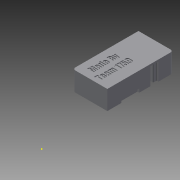
# Autodesk Inventor part: Positive Cap 535
Saved by Autodesk Inventor 2015 (Build 190159000, 159)
## iProperties
Created: 2015-01-23
Part Number: Positive Cap 535
Material: Generic
Document SubType Name: Modeling
Designer: pltwe4
Density: 1 g/cm^3
Appearance: Default
Author: pltwe4
Autodesk Inventor part; units mm, degrees
ref_plane "YZ Plane" through (0, 0, 0) normal (1, 0, 0) x (0, 1, 0)
ref_plane "XZ Plane" through (0, 0, 0) normal (0, 1, 0) x (-1, 0, 0)
ref_plane "XY Plane" through (0, 0, 0) normal (0, 0, 1) x (1, 0, 0)
sketch "Sketch1" plane through (0, 0, 0) normal (0, 1, 0) x (-1, 0, 0)
  line L0 (0, 0) -> (24.5364, 0)
  line L1 (24.5364, 0) -> (24.5364, -46.5582)
  line L2 (24.5364, -46.5582) -> (0, -46.5582)
  line L3 (0, -46.5582) -> (0, 0)
  dimension "d0" = 46.5582
  dimension "d1" = 24.5364
  constraints: 8 end point, 2 parallel, 1 horizontal, 1 perpendicular
  measures "d0" distance of L0.end L1.end
  measures "d1" distance of L1.end L2.end
extrude "Extrusion1" add sketch "Sketch1" along normal blind 13.5382
sketch "Sketch2" plane through (0, 0, 0) normal (0, -1, 0) x (1, 0, 0)
  point P0 (0, 0)
fillet "Fillet1" radius 1.905 1 edges at (-24.5364, 6.7691, -46.5582)
fillet "Fillet2" radius 1.905 1 edges at (0, 6.7691, 0)
sketch "Sketch3" plane through (0, 0, 0) normal (0, -1, 0) x (1, 0, 0)
  line L0 (-1.905, 0) -> (-24.5364, 0) projected
  arc A0 (0, -1.905) -> (-1.905, 0) centre (-1.905, -1.905) ccw projected
  line L1 (0, -46.5582) -> (0, -1.905) projected
  line L2 (-22.6314, -46.5582) -> (0, -46.5582) projected
  arc A1 (-24.5364, -44.6532) -> (-22.6314, -46.5582) centre (-22.6314, -44.6532) ccw projected
  line L3 (-24.5364, 0) -> (-24.5364, -44.6532) projected
  line L4 (-2.54, -2.54) -> (-21.9964, -2.54)
  line L5 (-21.9964, -44.0182) -> (-2.54, -44.0182)
  line L6 (0, -12.9032) -> (-4.445, -12.9032)
  line L7 (-4.445, -16.0782) -> (0, -16.0782)
  line L8 (-2.54, -44.0182) -> (-2.54, -18.6182)
  line L9 (-2.54, -10.3632) -> (-2.54, -2.54)
  line L10 (-4.445, -12.9032) -> (-4.445, -10.3632)
  line L11 (-4.445, -10.3632) -> (-2.54, -10.3632)
  line L12 (-4.445, -16.0782) -> (-4.445, -18.6182)
  line L13 (-4.445, -18.6182) -> (-2.54, -18.6182)
  line L14 (-21.9964, -10.3632) -> (-18.4404, -10.3632)
  line L15 (-18.4404, -10.3632) -> (-18.4404, -18.6182)
  line L16 (-18.4404, -18.6182) -> (-21.9964, -18.6182)
  line L17 (-21.9964, -2.54) -> (-21.9964, -10.3632)
  line L18 (-21.9964, -18.6182) -> (-21.9964, -44.0182)
  line L19 (0, -14.4907) -> (-5.2569, -14.4907) construction
  line L20 (-4.445, -11.6332) -> (-18.4404, -11.6332)
  line L21 (-4.445, -17.3482) -> (-18.4404, -17.3482)
  point P0 (0, 0)
  dimension "d7" = 2.54
  dimension "d9" = 2.54
  dimension "d11" = 3.175
  dimension "d13" = 4.445
  dimension "d14" = 2.54
  dimension "d15" = 2.54
  dimension "d16" = 2.54
  dimension "d17" = 2.54
  dimension "d20" = 2.54
  dimension "d21" = 6.096
  dimension "d22" = 2.54
  dimension "d37" = 32.0675
  constraints: 36 end point, 9 perpendicular, 7 parallel, 5 point on line, 4 horizontal, 2 collinear, 2 midpoint, 2 vertical, 1 other
  measures "d7" distance between parallel lines of L0 L4
  measures "d9" distance between parallel lines of L2 L5
  measures "d11" distance between parallel lines of L6 L7
  measures "d13" distance between parallel lines of L1 L10
  measures "d14" distance of L7.start L12.end
  measures "d15" distance of L6.end L10.end
  measures "d16" distance between parallel lines of L1 L8
  measures "d17" distance between parallel lines of L1 L9
  measures "d20" distance between parallel lines of L3 L18
  measures "d21" distance between parallel lines of L3 L15
  measures "d22" distance between parallel lines of L3 L17
  measures "d37" distance between parallel lines of L2 L19
extrude "Extrusion2" cut sketch "Sketch3" against normal blind 12.2682 contours L1 L7 L12 L21 L15 L20 L10 L6 | L20 L15 L14 L17 L4 L9 L11 L10 | L12 L13 L8 L5 L18 L16 L15 L21
sketch "Sketch4" plane through (0, 12.2682, 0) normal (0, -1, 0) x (1, 0, 0)
  line L0 (-4.5974, -23.6982) -> (-17.2974, -23.6982)
  line L1 (-17.2974, -23.6982) -> (-17.2974, -35.1282)
  line L2 (-17.2974, -35.1282) -> (-4.5974, -35.1282)
  line L3 (-4.5974, -35.1282) -> (-4.5974, -23.6982)
  line L4 (-2.54, -44.0182) -> (-21.9964, -44.0182) projected
  line L5 (-2.54, -18.6182) -> (-2.54, -44.0182) projected
  line L6 (-10.9474, -23.6982) -> (-10.9474, -35.1282) construction
  line L7 (-24.5364, 0) -> (-24.5364, -44.6532) construction
  line L8 (-22.6314, -46.5582) -> (0, -46.5582) construction
  point P0 (0, 0)
  dimension "d23" = 13.589
  dimension "d24" = 12.7
  dimension "d25" = 11.43
  dimension "d26" = 22.86
  constraints: 10 end point, 2 midpoint, 2 parallel, 1 horizontal, 1 perpendicular
  measures "d23" distance between parallel lines of L7 L6
  measures "d24" distance between parallel lines of L1 L3
  measures "d25" distance between parallel lines of L0 L2
  measures "d26" distance between parallel lines of L8 L0
extrude "Extrusion3" add sketch "Sketch4" along normal up to surface (12.2682 mm away)
sketch "Sketch5" plane through (-4.5974, 12.2682, -35.1282) normal (0, 0, -1) x (-1, 0, 0)
  line L0 (0, 0) -> (0, -12.2682) projected
  line L1 (12.7, 0) -> (12.7, -12.2682) projected
  line L2 (12.7, -12.2682) -> (0, -12.2682) projected
  arc A0 (8.2396, -6.5778) -> (4.4604, -6.5778) centre (6.35, -5.1816) ccw
  line L3 (6.35, -12.2682) -> (6.35, 0) construction
  line L4 (17.399, 0) -> (-2.0574, 0) construction
  line L5 (8.2396, -6.5778) -> (8.4707, -7.62)
  line L6 (8.4707, -7.62) -> (11.0107, -7.62)
  line L7 (11.0107, -7.62) -> (12.7, 0)
  line L8 (4.4604, -6.5778) -> (4.2293, -7.62)
  line L9 (4.2293, -7.62) -> (1.6893, -7.62)
  line L10 (1.6893, -7.62) -> (0, 0)
  point P0 (-4.5974, -12.2682)
  dimension "d29" = 7.0866
  dimension "d30" = 4.699
  dimension "d32" = 7.62
  dimension "d33" = 2.54
  dimension "d36" = 25
  constraints: 14 end point, 2 horizontal, 2 point on circle, 2 point on line, 1 centre point, 1 equal length, 1 midpoint, 1 parallel, 1 vertical, 2 other
  measures "d29" distance from line of L2 A0.centre
  measures "d30" diameter of A0
  measures "d32" distance between parallel lines of L4 L6
  measures "d33" distance of L5.end L6.end
  measures "d36" angle of L5 L8
extrude "Extrusion4" cut sketch "Sketch5" against normal up to surface (11.43 mm away)
sketch "Sketch6" plane through (0, 12.2682, 0) normal (0, -1, 0) x (1, 0, 0)
  line L0 (-4.445, -10.3632) -> (-4.445, -12.9032) projected
  line L1 (-4.445, -16.0782) -> (-4.445, -18.6182) projected
  line L2 (-18.4404, -18.6182) -> (-18.4404, -10.3632) projected
  line L3 (0, -12.9032) -> (0, -16.0782) projected
  line L4 (0, -16.0782) -> (-4.445, -16.0782) projected
  line L5 (-4.445, -12.9032) -> (0, -12.9032) projected
  line L6 (-4.445, -10.3632) -> (-18.4404, -10.3632)
  line L7 (-18.4404, -18.6182) -> (-4.445, -18.6182)
  line L8 (-1.27, -12.9032) -> (-1.27, -16.0782)
  point P0 (0, 0)
  dimension "d46" = 1.27
  constraints: 6 end point, 2 point on line, 1 horizontal, 1 parallel, 1 perpendicular
  measures "d46" distance between parallel lines of L8 L3
extrude "Extrusion5" cut sketch "Sketch6" against normal blind 0.635
sketch "Sketch7" plane through (0, 0, 0) normal (0, -1, 0) x (1, 0, 0)
  line L0 (0, -12.9032) -> (0, -1.905) projected
  line L1 (0, -1.905) -> (0, -46.5582) projected
  line L2 (0, -10.3632) -> (-0.635, -10.3632)
  line L3 (-1.27, -10.9982) -> (-1.27, -12.2682)
  arc A0 (-0.635, -10.3632) -> (-1.27, -10.9982) centre (-0.635, -10.9982) ccw
  line L4 (-1.905, -12.9032) -> (-4.445, -12.9032)
  line L5 (-4.445, -10.3632) -> (-4.445, -12.9032) projected
  arc A1 (-1.905, -12.9032) -> (-1.27, -12.2682) centre (-1.905, -12.2682) ccw
  line L6 (0, -10.3632) -> (0, -12.9032)
  line L7 (0, -12.9032) -> (-1.905, -12.9032)
  line L8 (-4.445, -12.9032) -> (0, -12.9032) projected
  point P0 (0, 0)
  point P1 (-1.27, -10.3632)
  point P2 (-1.27, -12.9032)
  dimension "d40" = 1.27
  dimension "d41" = 2.54
  dimension "d42" = 0.635
  dimension "d43" = 0.635
  constraints: 10 end point, 5 point on line, 5 tangent, 4 point on circle, 2 centre point, 2 collinear, 2 perpendicular, 1 parallel
  measures "d40" distance of L2.start point (-1.27, -10.363)
  measures "d41" distance of point (-1.27, -10.363) point (-1.27, -12.903)
  measures "d42" radius of A0
  measures "d43" radius of A1
extrude "Extrusion7" add sketch "Sketch6" against normal blind 0.635 contours L5 L3 L4 L8
extrude "Extrusion8" cut sketch "Sketch7" against normal up to surface (12.2682 mm away)
sketch "Sketch8" plane through (0, 0, -46.5582) normal (1, 0, 0) x (0, 0, -1)
  line L0 (-36.195, 0) -> (-36.195, 12.2682) projected
  line L1 (-30.48, 12.2682) -> (-36.195, 12.2682) projected
  line L2 (-30.48, 12.2682) -> (-30.48, 0) projected
  line L3 (0, 0) -> (-30.48, 0) projected
  line L4 (0, 0) -> (0, 13.5382) projected
  line L5 (-44.6532, 13.5382) -> (0, 13.5382) projected
  line L6 (-44.6532, 0) -> (-44.6532, 13.5382) projected
  line L7 (-36.195, 0) -> (-44.6532, 0) projected
  line L8 (-22.5397, 0) -> (-22.5397, 2.54)
  line L9 (-22.5397, 2.54) -> (-9.8397, 2.54)
  line L10 (-9.8397, 2.54) -> (-9.8397, 0)
  point P0 (-46.5582, 0)
  dimension "d51" = 2.54
  dimension "d52" = 12.7
  constraints: 6 end point, 2 perpendicular, 2 point on line, 1 vertical
  measures "d51" distance of L9.end L10.end
  measures "d52" distance of L8.end L9.end
extrude "Extrusion9" cut sketch "Sketch8" against normal blind 1.27 contours L8 L9 L10 L3
sketch "Sketch9" plane through (-4.5974, 12.2682, -35.1282) normal (0, 0, -1) x (-1, 0, 0)
  line L0 (12.7, 0) -> (11.0107, -7.62) projected
  line L1 (11.0107, -7.62) -> (8.4707, -7.62) projected
  line L2 (8.4707, -7.62) -> (8.2396, -6.5778) projected
  arc A0 (8.2396, -6.5778) -> (4.4604, -6.5778) centre (6.35, -5.1816) ccw projected
  line L3 (4.4604, -6.5778) -> (4.2293, -7.62) projected
  line L4 (4.2293, -7.62) -> (1.6893, -7.62) projected
  line L5 (1.6893, -7.62) -> (0, 0) projected
  line L6 (12.7, 0) -> (0, 0) projected
  line L7 (1.6893, -7.62) -> (11.0107, -7.62)
  line L8 (4.2293, -7.62) -> (1.6893, -7.62) projected
  point P0 (-4.5974, -12.2682)
  constraints: 2 end point, 1 collinear
extrude "Extrusion10" add sketch "Sketch9" along normal blind 2.54
mirror "Mirror1" about plane through (0, 0, -46.5582) normal (0, 0, -1) remove original yes
sketch "Sketch10" plane through (-24.5364, 13.5382, -93.1164) normal (0, 1, 0) x (1, 0, 0)
  arc A0 (24.5364, -1.905) -> (22.6314, 0) centre (22.6314, -1.905) ccw projected
  line L0 (0, 0) -> (22.6314, 0) projected
  line L1 (0, -44.6532) -> (0, 0) projected
  arc A1 (0, -44.6532) -> (1.905, -46.5582) centre (1.905, -44.6532) ccw projected
  line L2 (24.5364, -46.5582) -> (1.905, -46.5582) projected
  line L3 (24.5364, -1.905) -> (24.5364, -46.5582) projected
  line L4 (4.9657, -44.5516) -> (4.9657, -19.1516) construction
  line L5 (4.9657, -19.1516) -> (17.6657, -19.1516) construction
  line L6 (17.6657, -19.1516) -> (17.6657, -44.5516) construction
  line L7 (17.6657, -44.5516) -> (4.9657, -44.5516) construction
  line L8 (0, -44.6532) -> (0, 0) construction
  line L9 (24.5364, -1.905) -> (24.5364, -46.5582) construction
  line L10 (22.6314, 0) -> (0, 0) construction
  line L11 (24.5364, -46.5582) -> (1.905, -46.5582) construction
  line L12 (4.9657, -31.8516) -> (17.6657, -31.8516) construction
  line L13 (11.3157, -44.5516) -> (11.3157, -19.1516) construction
  line L14 (0, -22.3266) -> (24.5364, -22.3266) construction
  line L15 (11.3157, 0) -> (11.3157, -46.5582) construction
  line L16 (4.9657, -37.7102) -> (9.4107, -37.7102)
  line L17 (9.4107, -37.7102) -> (9.4107, -38.7218)
  line L18 (9.4107, -38.7218) -> (6.4094, -38.7218)
  line L19 (6.4094, -38.7218) -> (9.4107, -39.1271)
  line L20 (9.4107, -39.1271) -> (9.4107, -39.8405)
  line L21 (9.4107, -39.8405) -> (6.4764, -40.2626)
  line L22 (6.4764, -40.2626) -> (9.4107, -40.2659)
  line L23 (9.4107, -40.2659) -> (9.4107, -41.2775)
  line L24 (9.4107, -41.2775) -> (4.9657, -41.2775)
  line L25 (4.9657, -41.2775) -> (4.9657, -39.7802)
  spline S0 degree 2 poles (4.9657, -39.7802) (5.3643, -39.7166) (5.9103, -39.6429) knots 0 0 0 1 1 1
  line L26 (5.9103, -39.6429) -> (7.0425, -39.4788)
  line L27 (7.0425, -39.4788) -> (4.9657, -39.2175)
  line L28 (4.9657, -39.2175) -> (4.9657, -37.7102)
  line L29 (7.1765, -36.2866) -> (7.1765, -37.3283)
  line L30 (7.1765, -37.3283) -> (6.932, -37.3283)
  spline S1 degree 2 poles (6.932, -37.3283) (6.5099, -37.3283) (6.051, -37.134) (5.6993, -36.5445) (5.6993, -36.0755) knots 0 0 0 1 2 3 3 3
  spline S2 degree 2 poles (5.6993, -36.0755) (5.6993, -35.5128) (6.0979, -34.94) (6.6774, -34.8261) (7.5818, -34.8261) knots 0 0 0 1 2 3 3 3
  line L31 (7.5818, -34.8261) -> (9.4107, -34.8261)
  line L32 (9.4107, -34.8261) -> (9.4107, -35.9047)
  line L33 (9.4107, -35.9047) -> (9.0858, -35.9047)
  spline S3 degree 2 poles (9.0858, -35.9047) (9.2801, -36.0052) (9.4777, -36.3267) (9.4777, -36.5512) knots 0 0 0 1 2 2 2
  spline S4 degree 2 poles (9.4777, -36.5512) (9.4777, -36.8426) (9.1494, -37.3283) (8.5967, -37.3283) knots 0 0 0 1 2 2 2
  line L34 (8.5967, -37.3283) -> (8.2986, -37.3283)
  spline S5 degree 2 poles (8.2986, -37.3283) (7.89, -37.3283) (7.5918, -37.0704) (7.3942, -36.5579) knots 0 0 0 1 2 2 2
  spline S6 degree 2 poles (7.3942, -36.5579) (7.1798, -36.0119) (7.0324, -35.9348) (6.8047, -35.9348) knots 0 0 0 1 2 2 2
  spline S7 degree 2 poles (6.8047, -35.9348) (6.5199, -35.9348) (6.3458, -36.0186) (6.3458, -36.1191) knots 0 0 0 1 2 2 2
  spline S8 degree 2 poles (6.3458, -36.1191) (6.3458, -36.233) (6.4898, -36.2866) (6.7946, -36.2866) knots 0 0 0 1 2 2 2
  line L35 (6.7946, -36.2866) -> (7.1765, -36.2866)
  spline S9 degree 2 poles (7.6756, -35.9348) (7.8699, -36.2028) (8.1345, -36.2866) (8.3824, -36.2866) knots 0 0 0 1 2 2 2
  spline S10 degree 2 poles (8.3824, -36.2866) (8.6671, -36.2866) (8.8312, -36.2129) (8.8312, -36.1023) knots 0 0 0 1 2 2 2
  spline S11 degree 2 poles (8.8312, -36.1023) (8.8312, -35.9985) (8.7006, -35.9348) (8.4259, -35.9348) knots 0 0 0 1 2 2 2
  line L36 (8.4259, -35.9348) -> (7.6756, -35.9348)
  line L37 (4.9657, -31.9219) -> (9.4107, -31.9219)
  line L38 (9.4107, -31.9219) -> (9.4107, -33.0307)
  line L39 (9.4107, -33.0307) -> (9.1461, -33.0307)
  spline S12 degree 2 poles (9.1461, -33.0307) (9.3136, -33.1915) (9.4777, -33.5398) (9.4777, -33.7341) knots 0 0 0 1 2 2 2
  spline S13 degree 2 poles (9.4777, -33.7341) (9.4777, -33.992) (9.2064, -34.3705) (8.848, -34.4777) (8.446, -34.4777) knots 0 0 0 1 2 3 3 3
  line L40 (8.446, -34.4777) -> (6.7377, -34.4777)
  spline S14 degree 2 poles (6.7377, -34.4777) (6.319, -34.4777) (5.9672, -34.3705) (5.6993, -33.9853) (5.6993, -33.7207) knots 0 0 0 1 2 3 3 3
  spline S15 degree 2 poles (5.6993, -33.7207) (5.6993, -33.513) (5.8467, -33.1714) (5.9974, -33.0307) knots 0 0 0 1 2 2 2
  line L41 (5.9974, -33.0307) -> (4.9657, -33.0307)
  line L42 (4.9657, -33.0307) -> (4.9657, -31.9219)
  spline S16 degree 2 poles (6.6841, -33.0307) (6.4831, -33.0307) (6.3458, -33.101) (6.3458, -33.2015) knots 0 0 0 1 2 2 2
  spline S17 degree 2 poles (6.3458, -33.2015) (6.3458, -33.2987) (6.4697, -33.369) (6.6841, -33.369) knots 0 0 0 1 2 2 2
  line L43 (6.6841, -33.369) -> (8.4694, -33.369)
  spline S18 degree 2 poles (8.4694, -33.369) (8.6905, -33.369) (8.8312, -33.302) (8.8312, -33.2082) knots 0 0 0 1 2 2 2
  spline S19 degree 2 poles (8.8312, -33.2082) (8.8312, -33.101) (8.6738, -33.0307) (8.369, -33.0307) knots 0 0 0 1 2 2 2
  line L44 (8.369, -33.0307) -> (6.6841, -33.0307)
  line L45 (7.6521, -29.0111) -> (7.6521, -30.4481)
  line L46 (7.6521, -30.4481) -> (8.4393, -30.4481)
  spline S20 degree 2 poles (8.4393, -30.4481) (8.6872, -30.4481) (8.8312, -30.3777) (8.8312, -30.2739) knots 0 0 0 1 2 2 2
  spline S21 degree 2 poles (8.8312, -30.2739) (8.8312, -30.1466) (8.6403, -30.0629) (8.369, -30.0629) knots 0 0 0 1 2 2 2
  line L47 (8.369, -30.0629) -> (7.89, -30.0629)
  line L48 (7.89, -30.0629) -> (7.89, -29.0111)
  line L49 (7.89, -29.0111) -> (8.1579, -29.0111)
  spline S22 degree 2 poles (8.1579, -29.0111) (8.4962, -29.0111) (8.858, -29.0948) (9.27, -29.4097) (9.4777, -29.8887) (9.4777, -30.2538) knots 0 0 0 1 2 3 4 4 4
  spline S23 degree 2 poles (9.4777, -30.2538) (9.4777, -30.6055) (9.2734, -31.1415) (8.9183, -31.4429) (8.4929, -31.5568) (8.0876, -31.5568) knots 0 0 0 1 2 3 4 4 4
  line L50 (8.0876, -31.5568) -> (7.0224, -31.5568)
  spline S24 degree 2 poles (7.0224, -31.5568) (6.5467, -31.5568) (5.994, -31.2989) (5.6993, -30.7094) (5.6993, -30.3309) knots 0 0 0 1 2 3 3 3
  spline S25 degree 2 poles (5.6993, -30.3309) (5.6993, -29.8619) (6.0543, -29.2556) (6.6372, -29.0111) (7.1698, -29.0111) knots 0 0 0 1 2 3 3 3
  line L51 (7.1698, -29.0111) -> (7.6521, -29.0111)
  line L52 (7.0592, -30.1232) -> (6.7946, -30.1232)
  spline S26 degree 2 poles (6.7946, -30.1232) (6.5099, -30.1232) (6.3458, -30.1835) (6.3458, -30.2773) knots 0 0 0 1 2 2 2
  spline S27 degree 2 poles (6.3458, -30.2773) (6.3458, -30.3945) (6.4864, -30.4481) (6.7946, -30.4481) knots 0 0 0 1 2 2 2
  line L53 (6.7946, -30.4481) -> (7.0592, -30.4481)
  line L54 (7.0592, -30.4481) -> (7.0592, -30.1232)
  line L55 (4.9657, -27.6243) -> (4.9657, -26.472)
  spline S28 degree 2 poles (4.9657, -26.472) (4.9657, -25.9227) (5.1365, -25.36) (5.6557, -25.0149) (6.2319, -25.0149) knots 0 0 0 1 2 3 3 3
  spline S29 degree 2 poles (6.2319, -25.0149) (6.6204, -25.0149) (6.9286, -25.2595) (7.009, -25.6212) knots 0 0 0 1 2 2 2
  spline S30 degree 2 poles (7.009, -25.6212) (7.1028, -25.2193) (7.5215, -24.9346) (7.9569, -24.9346) knots 0 0 0 1 2 2 2
  line L56 (7.9569, -24.9346) -> (8.3656, -24.9346)
  spline S31 degree 2 poles (8.3656, -24.9346) (8.8178, -24.9346) (9.2499, -25.1389) (9.4107, -25.5911) (9.4107, -26.2878) knots 0 0 0 1 2 3 3 3
  line L57 (9.4107, -26.2878) -> (9.4107, -27.6243)
  line L58 (9.4107, -27.6243) -> (4.9657, -27.6243)
  line L59 (7.4076, -26.4687) -> (8.6503, -26.4687)
  spline S32 degree 2 poles (8.6503, -26.4687) (8.6436, -26.2242) (8.5063, -26.0902) (8.235, -26.0902) knots 0 0 0 1 2 2 2
  line L60 (8.235, -26.0902) -> (7.823, -26.0902)
  spline S33 degree 2 poles (7.823, -26.0902) (7.5349, -26.0902) (7.4143, -26.2108) (7.4076, -26.4687) knots 0 0 0 1 2 2 2
  line L61 (5.7261, -26.4687) -> (6.7142, -26.4687)
  spline S34 degree 2 poles (6.7142, -26.4687) (6.7109, -26.395) (6.7109, -26.3548) knots 0 0 0 1 1 1
  spline S35 degree 2 poles (6.7109, -26.3548) (6.7109, -26.184) (6.5434, -26.0902) (6.1481, -26.0902) knots 0 0 0 1 2 2 2
  spline S36 degree 2 poles (6.1481, -26.0902) (5.9405, -26.0902) (5.773, -26.1672) (5.7294, -26.2912) (5.7261, -26.4687) knots 0 0 0 1 2 3 3 3
  line L62 (5.7663, -22.228) -> (8.4025, -22.5462)
  spline S37 degree 2 poles (8.4025, -22.5462) (9.0288, -22.6233) (9.4844, -22.7238) (9.7792, -22.9583) (9.9198, -23.3803) (9.9198, -23.8426) knots 0 0 0 1 2 3 4 4 4
  line L63 (9.9198, -23.8426) -> (9.9198, -24.5158)
  line L64 (9.9198, -24.5158) -> (9.337, -24.5158)
  spline S38 degree 2 poles (9.337, -24.5158) (9.337, -24.2546) (9.2834, -24.1072) (9.193, -24.1072) knots 0 0 0 1 2 2 2
  spline S39 degree 2 poles (9.193, -24.1072) (9.1494, -24.1072) (8.8111, -24.1742) knots 0 0 0 1 1 1
  line L65 (8.8111, -24.1742) -> (5.7663, -24.7838)
  line L66 (5.7663, -24.7838) -> (5.7663, -23.7756)
  line L67 (5.7663, -23.7756) -> (8.2283, -23.4105)
  line L68 (8.2283, -23.4105) -> (5.7663, -23.2363)
  line L69 (5.7663, -23.2363) -> (5.7663, -22.228)
  line L70 (12.4044, -41.3094) -> (13.2955, -41.3094)
  line L71 (13.2955, -41.3094) -> (13.2955, -41.996)
  line L72 (13.2955, -41.996) -> (16.8494, -41.996)
  line L73 (16.8494, -41.996) -> (16.8494, -43.1517)
  line L74 (16.8494, -43.1517) -> (13.2955, -43.1517)
  line L75 (13.2955, -43.1517) -> (13.2955, -43.835)
  line L76 (13.2955, -43.835) -> (12.4044, -43.835)
  line L77 (12.4044, -43.835) -> (12.4044, -41.3094)
  line L78 (15.0909, -38.566) -> (15.0909, -40.003)
  line L79 (15.0909, -40.003) -> (15.878, -40.003)
  spline S40 degree 2 poles (15.878, -40.003) (16.1259, -40.003) (16.27, -39.9327) (16.27, -39.8288) knots 0 0 0 1 2 2 2
  spline S41 degree 2 poles (16.27, -39.8288) (16.27, -39.7015) (16.079, -39.6178) (15.8077, -39.6178) knots 0 0 0 1 2 2 2
  line L80 (15.8077, -39.6178) -> (15.3287, -39.6178)
  line L81 (15.3287, -39.6178) -> (15.3287, -38.566)
  line L82 (15.3287, -38.566) -> (15.5967, -38.566)
  spline S42 degree 2 poles (15.5967, -38.566) (15.935, -38.566) (16.2968, -38.6497) (16.7088, -38.9646) (16.9164, -39.4436) (16.9164, -39.8087) knots 0 0 0 1 2 3 4 4 4
  spline S43 degree 2 poles (16.9164, -39.8087) (16.9164, -40.1604) (16.7121, -40.6964) (16.357, -40.9978) (15.9316, -41.1117) (15.5263, -41.1117) knots 0 0 0 1 2 3 4 4 4
  line L83 (15.5263, -41.1117) -> (14.4611, -41.1117)
  spline S44 degree 2 poles (14.4611, -41.1117) (13.9855, -41.1117) (13.4328, -40.8538) (13.138, -40.2643) (13.138, -39.8858) knots 0 0 0 1 2 3 3 3
  spline S45 degree 2 poles (13.138, -39.8858) (13.138, -39.4168) (13.4931, -38.8105) (14.0759, -38.566) (14.6085, -38.566) knots 0 0 0 1 2 3 3 3
  line L84 (14.6085, -38.566) -> (15.0909, -38.566)
  line L85 (14.498, -39.6781) -> (14.2334, -39.6781)
  spline S46 degree 2 poles (14.2334, -39.6781) (13.9486, -39.6781) (13.7845, -39.7384) (13.7845, -39.8322) knots 0 0 0 1 2 2 2
  spline S47 degree 2 poles (13.7845, -39.8322) (13.7845, -39.9494) (13.9252, -40.003) (14.2334, -40.003) knots 0 0 0 1 2 2 2
  line L86 (14.2334, -40.003) -> (14.498, -40.003)
  line L87 (14.498, -40.003) -> (14.498, -39.6781)
  line L88 (14.6152, -37.2127) -> (14.6152, -38.2545)
  line L89 (14.6152, -38.2545) -> (14.3707, -38.2545)
  spline S48 degree 2 poles (14.3707, -38.2545) (13.9486, -38.2545) (13.4897, -38.0602) (13.138, -37.4707) (13.138, -37.0017) knots 0 0 0 1 2 3 3 3
  spline S49 degree 2 poles (13.138, -37.0017) (13.138, -36.439) (13.5366, -35.8662) (14.1161, -35.7523) (15.0205, -35.7523) knots 0 0 0 1 2 3 3 3
  line L90 (15.0205, -35.7523) -> (16.8494, -35.7523)
  line L91 (16.8494, -35.7523) -> (16.8494, -36.8309)
  line L92 (16.8494, -36.8309) -> (16.5245, -36.8309)
  spline S50 degree 2 poles (16.5245, -36.8309) (16.7188, -36.9314) (16.9164, -37.2529) (16.9164, -37.4774) knots 0 0 0 1 2 2 2
  spline S51 degree 2 poles (16.9164, -37.4774) (16.9164, -37.7688) (16.5882, -38.2545) (16.0355, -38.2545) knots 0 0 0 1 2 2 2
  line L93 (16.0355, -38.2545) -> (15.7374, -38.2545)
  spline S52 degree 2 poles (15.7374, -38.2545) (15.3287, -38.2545) (15.0306, -37.9966) (14.833, -37.4841) knots 0 0 0 1 2 2 2
  spline S53 degree 2 poles (14.833, -37.4841) (14.6186, -36.9381) (14.4712, -36.861) (14.2434, -36.861) knots 0 0 0 1 2 2 2
  spline S54 degree 2 poles (14.2434, -36.861) (13.9587, -36.861) (13.7845, -36.9448) (13.7845, -37.0452) knots 0 0 0 1 2 2 2
  spline S55 degree 2 poles (13.7845, -37.0452) (13.7845, -37.1591) (13.9285, -37.2127) (14.2334, -37.2127) knots 0 0 0 1 2 2 2
  line L94 (14.2334, -37.2127) -> (14.6152, -37.2127)
  spline S56 degree 2 poles (15.1143, -36.861) (15.3086, -37.129) (15.5732, -37.2127) (15.8211, -37.2127) knots 0 0 0 1 2 2 2
  spline S57 degree 2 poles (15.8211, -37.2127) (16.1058, -37.2127) (16.27, -37.139) (16.27, -37.0285) knots 0 0 0 1 2 2 2
  spline S58 degree 2 poles (16.27, -37.0285) (16.27, -36.9247) (16.1393, -36.861) (15.8646, -36.861) knots 0 0 0 1 2 2 2
  line L95 (15.8646, -36.861) -> (15.1143, -36.861)
  line L96 (13.205, -34.2751) -> (13.5534, -34.2952)
  spline S59 degree 2 poles (13.5534, -34.2952) (13.3457, -34.1645) (13.138, -33.8095) (13.138, -33.5817) knots 0 0 0 1 2 2 2
  spline S60 degree 2 poles (13.138, -33.5817) (13.138, -33.1362) (13.5534, -32.8816) knots 0 0 0 1 1 1
  spline S61 degree 2 poles (13.5534, -32.8816) (13.3457, -32.7409) (13.138, -32.3892) (13.138, -32.1748) knots 0 0 0 1 2 2 2
  spline S62 degree 2 poles (13.138, -32.1748) (13.138, -31.8935) (13.4127, -31.5217) (13.8113, -31.4178) (14.2602, -31.4178) knots 0 0 0 1 2 3 3 3
  line L97 (14.2602, -31.4178) -> (16.8494, -31.4178)
  line L98 (16.8494, -31.4178) -> (16.8494, -32.4931)
  line L99 (16.8494, -32.4931) -> (14.4745, -32.4931)
  spline S63 degree 2 poles (14.4745, -32.4931) (14.0056, -32.4931) (13.7845, -32.5567) (13.7845, -32.6706) knots 0 0 0 1 2 2 2
  spline S64 degree 2 poles (13.7845, -32.6706) (13.7845, -32.7912) (14.0056, -32.8582) (14.4745, -32.8582) knots 0 0 0 1 2 2 2
  line L100 (14.4745, -32.8582) -> (16.8494, -32.8582)
  line L101 (16.8494, -32.8582) -> (16.8494, -33.9334)
  line L102 (16.8494, -33.9334) -> (14.5348, -33.9334)
  spline S65 degree 2 poles (14.5348, -33.9334) (13.9989, -33.9334) (13.7845, -33.987) (13.7845, -34.1042) knots 0 0 0 1 2 2 2
  spline S66 degree 2 poles (13.7845, -34.1042) (13.7845, -34.1779) (13.8984, -34.2851) (14.0592, -34.2952) (14.3238, -34.2952) knots 0 0 0 1 2 3 3 3
  line L103 (14.3238, -34.2952) -> (16.8494, -34.2952)
  line L104 (16.8494, -34.2952) -> (16.8494, -35.3704)
  line L105 (16.8494, -35.3704) -> (13.205, -35.3704)
  line L106 (13.205, -35.3704) -> (13.205, -34.2751)
  line L107 (12.4044, -28.3328) -> (16.8494, -28.3328)
  line L108 (16.8494, -28.3328) -> (16.8494, -29.4415)
  line L109 (16.8494, -29.4415) -> (14.4645, -29.4415)
  spline S67 degree 2 poles (14.4645, -29.4415) (13.9486, -29.4415) (13.741, -29.4918) (13.6338, -29.7128) (13.6338, -30.0947) knots 0 0 0 1 2 3 3 3
  line L110 (13.6338, -30.0947) -> (13.6338, -30.2052)
  line L111 (13.6338, -30.2052) -> (13.1146, -30.2052)
  spline S68 degree 2 poles (13.1146, -30.2052) (12.9437, -29.4013) (12.4044, -28.9826) knots 0 0 0 1 1 1
  line L112 (12.4044, -28.9826) -> (12.4044, -28.3328)
  line L113 (12.4044, -25.9445) -> (13.3759, -25.9445)
  line L114 (13.3759, -25.9445) -> (16.8494, -26.6513)
  line L115 (16.8494, -26.6513) -> (16.8494, -27.7566)
  line L116 (16.8494, -27.7566) -> (13.205, -26.9661)
  line L117 (13.205, -26.9661) -> (13.205, -28.0648)
  line L118 (13.205, -28.0648) -> (12.4044, -28.0648)
  line L119 (12.4044, -28.0648) -> (12.4044, -25.9445)
  line L120 (12.4044, -23.2781) -> (13.1146, -23.2781)
  line L121 (13.1146, -23.2781) -> (13.1146, -24.6549)
  line L122 (13.1146, -24.6549) -> (13.8716, -24.6549)
  spline S69 degree 2 poles (13.8716, -24.6549) (13.5668, -24.3969) (13.5668, -23.9883) knots 0 0 0 1 1 1
  spline S70 degree 2 poles (13.5668, -23.9883) (13.5668, -23.5294) (14.0793, -23.0604) (14.8095, -23.0604) knots 0 0 0 1 2 2 2
  line L123 (14.8095, -23.0604) -> (15.4426, -23.0604)
  spline S71 degree 2 poles (15.4426, -23.0604) (15.9149, -23.0604) (16.357, -23.1509) (16.7322, -23.449) (16.9332, -23.9782) (16.9332, -24.3601) knots 0 0 0 1 2 3 4 4 4
  spline S72 degree 2 poles (16.9332, -24.3601) (16.9332, -24.7888) (16.6351, -25.442) (16.0422, -25.7167) (15.4225, -25.7167) knots 0 0 0 1 2 3 3 3
  line L124 (15.4225, -25.7167) -> (15.1813, -25.7167)
  line L125 (15.1813, -25.7167) -> (15.1813, -24.608)
  line L126 (15.1813, -24.608) -> (15.4593, -24.608)
  spline S73 degree 2 poles (15.4593, -24.608) (15.8881, -24.608) (16.2499, -24.5477) (16.2499, -24.3668) knots 0 0 0 1 2 2 2
  spline S74 degree 2 poles (16.2499, -24.3668) (16.2499, -24.2864) (16.146, -24.1826) (16.0254, -24.1759) (15.5598, -24.1692) knots 0 0 0 1 2 3 3 3
  line L127 (15.5598, -24.1692) -> (14.6822, -24.1692)
  spline S75 degree 2 poles (14.6822, -24.1692) (14.431, -24.1692) (14.2501, -24.273) (14.2501, -24.3969) knots 0 0 0 1 2 2 2
  spline S76 degree 2 poles (14.2501, -24.3969) (14.2501, -24.474) (14.3439, -24.5778) (14.4511, -24.608) (14.6454, -24.608) knots 0 0 0 1 2 3 3 3
  line L128 (14.6454, -24.608) -> (14.6454, -25.7066)
  line L129 (14.6454, -25.7066) -> (12.4044, -25.6598)
  line L130 (12.4044, -25.6598) -> (12.4044, -23.2781)
  line L131 (15.667, -22.6819) -> (15.667, -21.5732)
  spline S77 degree 2 poles (15.667, -21.5732) (15.9785, -21.5732) (16.1393, -21.5564) (16.2499, -21.4392) (16.2499, -21.3353) knots 0 0 0 1 2 3 3 3
  spline S78 degree 2 poles (16.2499, -21.3353) (16.2499, -21.2516) (16.146, -21.1411) (15.9819, -21.1277) (15.7307, -21.1277) knots 0 0 0 1 2 3 3 3
  line L132 (15.7307, -21.1277) -> (15.0205, -21.1277)
  spline S79 degree 2 poles (15.0205, -21.1277) (15.1981, -21.2114) (15.3789, -21.5397) (15.3789, -21.7842) knots 0 0 0 1 2 2 2
  spline S80 degree 2 poles (15.3789, -21.7842) (15.3789, -22.089) (15.0507, -22.5546) (14.5884, -22.6819) (14.1965, -22.6819) knots 0 0 0 1 2 3 3 3
  line L133 (14.1965, -22.6819) -> (13.8415, -22.6819)
  spline S81 degree 2 poles (13.8415, -22.6819) (13.3759, -22.6819) (12.9203, -22.6082) (12.5317, -22.3) (12.3174, -21.7574) (12.3174, -21.3956) knots 0 0 0 1 2 3 4 4 4
  spline S82 degree 2 poles (12.3174, -21.3956) (12.3174, -20.9535) (12.5652, -20.3807) (13.0275, -20.0692) (13.54, -20.0189) (14.2736, -20.0189) knots 0 0 0 1 2 3 4 4 4
  line L134 (14.2736, -20.0189) -> (14.8899, -20.0189)
  spline S83 degree 2 poles (14.8899, -20.0189) (15.6838, -20.0189) (16.2197, -20.0625) (16.6987, -20.4008) (16.9365, -20.9769) (16.9365, -21.3554) knots 0 0 0 1 2 3 4 4 4
  spline S84 degree 2 poles (16.9365, -21.3554) (16.9365, -21.8244) (16.6351, -22.4206) (16.0857, -22.6819) (15.667, -22.6819) knots 0 0 0 1 2 3 3 3
  spline S85 degree 2 poles (14.2803, -21.5732) (14.5616, -21.5732) (14.6923, -21.4258) (14.6923, -21.3487) knots 0 0 0 1 2 2 2
  spline S86 degree 2 poles (14.6923, -21.3487) (14.6923, -21.2348) (14.5248, -21.1277) (14.2803, -21.1277) knots 0 0 0 1 2 2 2
  line L135 (14.2803, -21.1277) -> (13.4763, -21.1277)
  spline S87 degree 2 poles (13.4763, -21.1277) (13.1816, -21.1277) (13.0007, -21.2282) (13.0007, -21.3487) knots 0 0 0 1 2 2 2
  spline S88 degree 2 poles (13.0007, -21.3487) (13.0007, -21.4191) (13.1414, -21.5732) (13.4495, -21.5732) knots 0 0 0 1 2 2 2
  line L136 (13.4495, -21.5732) -> (14.2803, -21.5732)
  point P0 (24.5364, -93.1164)
  dimension "d57" = 25.4
  dimension "d58" = 12.7
  dimension "d60" = 9.525
  constraints: 8 end point, 6 midpoint, 2 perpendicular, 2 point on line, 1 collinear, 2 other
  measures "d57" distance of L4.start L4.end
  measures "d58" distance of L4.end L5.end
  measures "d60" distance between parallel lines of L14 L12
extrude "Extrusion11" cut sketch "Sketch10" against normal blind 0.635 contours L16 L17 L18 L19 L20 L21 L22 L23 L24 L25 S0 L26 L27 L28 | L29 L30 S1 S2 L31 L32 L33 S3 S4 L34 S5 S6 S7 S8 L35 | L37 L38 L39 S12 S13 L40 S14 S15 L41 L42 | L45 L46 S20 S21 L47 L48 L49 S22 S23 L50 S24 S25 L51 | L55 S28 S29 S30 L56 S31 L57 L58 | L62 S37 L63 L64 S38 S39 L65 L66 L67 L68 L69 | L70 L71 L72 L73 L74 L75 L76 L77 | L78 L79 S40 S41 L80 L81 L82 S42 S43 L83 S44 S45 L84 | L88 L89 S48 S49 L90 L91 L92 S50 S51 L93 S52 S53 S54 S55 L94 | L96 S59 S60 S61 S62 L97 L98 L99 S63 S64 L100 L101 L102 S65 S66 L103 L104 L105 L106 | L107 L108 L109 S67 L110 L111 S68 L112 | L113 L114 L115 L116 L117 L118 L119 | L120 L121 L122 S69 S70 L123 S71 S72 L124 L125 L126 S73 S74 L127 S75 S76 L128 L129 L130 | L131 S77 S78 L132 S79 S80 L133 S81 S82 L134 S83 S84
equation "\"d27\" = d2"
equation "\"d34\" = d2"
equation "\"d2\" = 13.5382"
body "Solid1"
